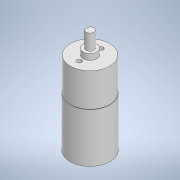
# Autodesk Inventor part: Stirring motor
Saved by Autodesk Inventor 2022 (Build 260153000, 153)
## iProperties
Created: 2022-06-22
Part Number: Stirring motor
Material: Generic
Document SubType Name: Modeling
Designer: efred
Density: 1 g/cm^3
Appearance: Default
Author: efred
Autodesk Inventor part; units mm, degrees
ref_plane "YZ Plane" through (0, 0, 0) normal (1, 0, 0) x (0, 1, 0)
ref_plane "XZ Plane" through (0, 0, 0) normal (0, 1, 0) x (-1, 0, 0)
ref_plane "XY Plane" through (0, 0, 0) normal (0, 0, 1) x (1, 0, 0)
sketch "Sketch1" plane through (0, 0, 0) normal (0, 1, 0) x (-1, 0, 0)
  circle A0 centre (0, 0) radius 10.2
  dimension "d0" = 20.4
  constraints: 1 centre point, 1 coincident
  measures "d0" diameter of A0
extrude "Extrusion1" add sketch "Sketch1" along normal blind 25.1
sketch "Sketch2" plane through (0, 25.1, 0) normal (0, 1, 0) x (1, 0, 0)
  circle A0 centre (0, 0) radius 10
  dimension "d3" = 20
  constraints: 1 centre point, 1 coincident
  measures "d3" diameter of A0
extrude "Extrusion2" add sketch "Sketch2" along normal blind 17
sketch "Sketch3" plane through (0, 42.1, 0) normal (0, 1, 0) x (1, 0, 0)
  circle A0 centre (0, 0) radius 3.5
  dimension "d6" = 7
  constraints: 1 centre point, 1 coincident
  measures "d6" diameter of A0
extrude "Extrusion3" add sketch "Sketch3" along normal blind 3
sketch "Sketch4" plane through (0, 45.1, 0) normal (0, 1, 0) x (1, 0, 0)
  circle A0 centre (0, 0) radius 10 projected
  circle A1 centre (0, 0) radius 2
  dimension "d9" = 4
  constraints: 1 centre point, 1 coincident
  measures "d9" diameter of A1
extrude "Extrusion4" add sketch "Sketch4" along normal blind 8 contours A1
sketch "Sketch5" plane through (0, 53.1, 0) normal (0, 1, 0) x (1, 0, 0)
  circle A0 centre (0, 0) radius 2 projected
  circle A1 centre (0, 0) radius 2 projected
  line L0 (-1.5, -1.3229) -> (-1.5, 1.3229)
  point P0 (-2, 0)
  dimension "d12" = 0.5
  constraints: 3 point on circle, 2 end point, 1 horizontal alignment, 1 vertical
  measures "d12" distance from line of L0 point (-2, 0)
extrude "Extrusion5" cut sketch "Sketch5" against normal blind 7 contours L0 A0 picked at (-1.5908, -0.3089)
sketch "Sketch6" plane through (0, 42.1, 0) normal (0, 1, 0) x (1, 0, 0)
  circle A0 centre (0, 5.5) radius 1.25
  line L0 (0, 0) -> (3.5, 0) construction
  circle A1 centre (0, 0) radius 3.5 projected
  circle A2 centre (0, -5.5) radius 1.25
  dimension "d15" = 2.5
  dimension "d16" = 11
  constraints: 2 centre point, 2 end point, 1 horizontal, 1 horizontal alignment, 1 symmetric about line, 1 vertical alignment, 2 other
  measures "d15" diameter of A0
  measures "d16" distance of A2.centre A0.centre
extrude "Extrusion6" cut sketch "Sketch6" against normal blind 10 contours A0 | A2
body "Solid1"
